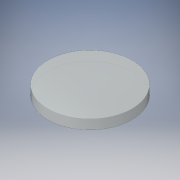
# Autodesk Inventor part: Track v3 Cover
Saved by Autodesk Inventor 2016 (Build 200138000, 138)
## iProperties
Created: 2016-05-24
Part Number: Track v3 Cover
Material: Glass
Document SubType Name: Modeling
Designer: xdlea
Density: 2.18 g/cm^3
Appearance: Clear
Author: xdlea
Autodesk Inventor part; units mm, degrees
ref_plane "YZ Plane" through (0, 0, 0) normal (1, 0, 0) x (0, 1, 0)
ref_plane "XZ Plane" through (0, 0, 0) normal (0, 1, 0) x (-1, 0, 0)
ref_plane "XY Plane" through (0, 0, 0) normal (0, 0, 1) x (1, 0, 0)
sketch "Sketch1" plane through (0, 0, 0) normal (0, 1, 0) x (-1, 0, 0)
  circle A0 centre (0, 0) radius 27.94
  dimension "d0" = 55.88
  constraints: 1 centre point, 1 coincident
  measures "d0" diameter of A0
extrude "Extrusion1" add sketch "Sketch1" along normal blind 6.35
body "Solid1"
